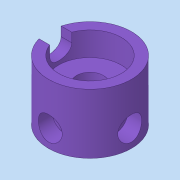
# Autodesk Inventor part: SpoolCarrageMagnetMountREV2
Saved by Autodesk Inventor 2017.3 (Build 213256000, 256)
## iProperties
Created: 2019-01-08
Part Number: SpoolCarrageMagnetMountREV2
Material: ABS Plastic
Document SubType Name: Modeling
Designer: Derek Wider
Density: 1.06 g/cm^3
Appearance: Violet
Author: Derek Wider
Autodesk Inventor part; units mm, degrees
ref_plane "XZ Plane" through (0, 0, 0) normal (0, 1, 0) x (-1, 0, 0)
ref_plane "XY Plane" through (0, 0, 0) normal (0, 0, 1) x (1, 0, 0)
sketch "Sketch1" plane through (0, 0, 0) normal (0, 1, 0) x (-1, 0, 0)
  circle A0 centre (0, 0) radius 4.318
  circle A1 centre (0, 0) radius 5.715
  dimension "d0" = 8.636
  dimension "d1" = 11.43
  constraints: 2 centre point, 2 coincident
  measures "d0" diameter of A0
  measures "d1" diameter of A1
extrude "Extrusion1" add sketch "Sketch1" along normal blind 3.302
sketch "Sketch2" plane through (0, 0, 0) normal (0, -1, 0) x (1, 0, 0)
  circle A0 centre (0, 0) radius 5.715 projected
  circle A1 centre (0, 0) radius 1.8415
  dimension "d4" = 3.683
  constraints: 1 centre point, 1 coincident
  measures "d4" diameter of A1
extrude "Extrusion2" add sketch "Sketch2" along normal blind 4.953
ref_plane "Work Plane1" through (-5.715, 0, 0) normal (1, 0, 0) x (0, 1, 0)
sketch "Sketch3" plane through (-5.715, 0, 0) normal (1, 0, 0) x (0, 1, 0)
  circle A0 centre (-2.54, 0) radius 1.651
  line L0 (-4.953, 5.715) -> (-4.953, -5.715) projected
  point P0 (0, 0)
  dimension "d7" = 3.302
  dimension "d8" = 2.413
  constraints: 1 centre point
  measures "d7" diameter of A0
  measures "d8" distance from line of L0 A0.centre
extrude "Extrusion3" cut sketch "Sketch3" along normal blind 2.159
pattern_circular "Circular Pattern1" count 4 over 360 about axis through (0, 0, 0) along (0, 1, 0) of "Extrusion3"
ref_plane "Work Plane2" through (-5.715, 0, 0) normal (1, 0, 0) x (0, 1, 0)
sketch "Sketch4" plane through (-5.715, 0, 0) normal (1, 0, 0) x (0, 1, 0)
  circle A0 centre (2.032, 0) radius 1.524
  line L0 (3.302, -5.715) -> (3.302, 5.715) projected
  line L1 (2.032, -1.524) -> (3.302, -1.524)
  line L2 (2.032, 1.524) -> (3.302, 1.524)
  point P0 (0, 0)
  dimension "d14" = 3.048
  dimension "d15" = 1.27
  constraints: 4 end point, 2 point on circle, 2 point on line, 2 tangent, 1 centre point, 1 horizontal, 1 perpendicular
  measures "d14" diameter of A0
  measures "d15" distance from line of A0.centre L0
extrude "Extrusion4" cut sketch "Sketch4" along normal blind 2.159 contours A0 L0 | L2 L0 A0 | A0 L0 L1 picked at (2.3744, -0.0612)
body "Solid1"
